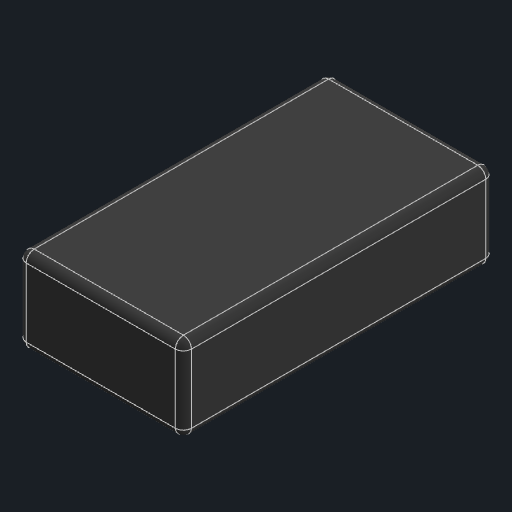
# Autodesk Inventor part: accumulators_case
Saved by Autodesk Inventor 2023 (Build 270158030, 158C)
## iProperties
Created: 2022-07-13
Part Number: accumulators_case
Material: Rubber, Silicone
Document SubType Name: Modeling
Designer: Norbert Ligas
Density: 1.25 g/cm^3
Appearance: Rubber - Black
batteries_case_width: 41,000 mm
batteries_case_length: 77,000 mm
batteries_case_height: 21,000 mm
Author: Norbert Ligas
Autodesk Inventor part; units mm, degrees
ref_plane "YZ Plane" through (0, 0, 0) normal (1, 0, 0) x (0, 1, 0)
ref_plane "XZ Plane" through (0, 0, 0) normal (0, 1, 0) x (-1, 0, 0)
ref_plane "XY Plane" through (0, 0, 0) normal (0, 0, 1) x (1, 0, 0)
sketch "Sketch1" plane through (0, 0, 0) normal (0, 1, 0) x (-1, 0, 0)
  line L0 (-20.5, -38.5) -> (20.5, -38.5)
  line L1 (20.5, -38.5) -> (20.5, 38.5)
  line L2 (20.5, 38.5) -> (-20.5, 38.5)
  line L3 (-20.5, 38.5) -> (-20.5, -38.5)
  line L4 (-20.5, -38.5) -> (20.5, 38.5) construction
  line L5 (20.5, -38.5) -> (-20.5, 38.5) construction
  point P0 (0, 0)
  dimension "d0" = 77
  dimension "d1" = 41
  constraints: 12 end point, 2 midpoint, 2 parallel, 1 horizontal, 1 perpendicular
  measures "d0" distance of L2.end L0.start
  measures "d1" distance of L0.start L0.end
extrude "Extrusion1" add sketch "Sketch1" along normal blind 21
fillet "Fillet1" radius 2 12 edges at (-20.5, 21, 0) (0, 21, 38.5) (-20.5, 10.5, 38.5) (0, 0, 38.5) (20.5, 10.5, 38.5) (20.5, 21, 0) (20.5, 0, 0) (20.5, 10.5, -38.5) (0, 0, -38.5) (0, 21, -38.5) (-20.5, 10.5, -38.5) (-20.5, 0, 0)
equation "\"d0\" = batteries_case_length"
equation "\"d1\" = batteries_case_width"
equation "\"d2\" = batteries_case_height"
equation "\"batteries_case_width\" = 41"
equation "\"batteries_case_length\" = 77"
equation "\"batteries_case_height\" = 21"
body "Solid1"
